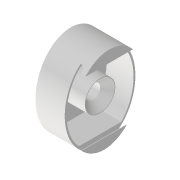
# Autodesk Inventor part: Spectrometer_pinholeholder_v0
Saved by Autodesk Inventor 2022 (Build 260153000, 153)
## iProperties
Created: 2023-02-14
Part Number: Spectrometer_pinholeholder_v0
Material: Generisch
Document SubType Name: Modeling
Designer: diederichbenedict
Density: 1 g/cm^3
Appearance: Vorgabe
Author: diederichbenedict
Autodesk Inventor part; units mm, degrees
ref_plane "YZ Plane" through (0, 0, 0) normal (1, 0, 0) x (0, 1, 0)
ref_plane "XZ Plane" through (0, 0, 0) normal (0, 1, 0) x (-1, 0, 0)
ref_plane "XY Plane" through (0, 0, 0) normal (0, 0, 1) x (1, 0, 0)
sketch "Skizze1" plane through (0, 0, 0) normal (0, 0, 1) x (1, 0, 0)
  line L0 (0, -2.5771) -> (1.4822, -3.4328)
  line L1 (-1, -2.5771) -> (0, -2.5771)
  line L2 (-1, -2.5771) -> (-1, -5.866)
  arc A0 (-1, -5.866) -> (-0.067, -6.116) centre (-0.5, -5.866) ccw
  line L3 (-0.067, -6.116) -> (1.4822, -3.4328)
  line L4 (1.6163, 54.0505) -> (2.3924, 51.1542)
  spline S0 degree 3 poles (3.0047, 50.8006) (2.979, 50.7937) (2.9516, 50.7885) (2.8832, 50.7821) (2.8365, 50.7824) (2.7601, 50.7963) (2.7337, 50.8032) (2.6799, 50.8225) (2.6525, 50.8349) (2.6004, 50.865) (2.5753, 50.8826) (2.5312, 50.9197) (2.5121, 50.9392) (2.4385, 51.0245) (2.4075, 51.0976) (2.3924, 51.1542) knots 0 0 0 0 0.142019 0.142019 0.325993 0.325993 0.417981 0.417981 0.509968 0.509968 0.59446 0.59446 0.678952 0.678952 1 1 1 1
  line L5 (3.0047, 50.8006) -> (6.1012, 51.6303)
  spline S1 degree 3 poles (1.6163, 54.0505) (1.5827, 54.1758) (1.4869, 54.2944) (1.3833, 54.3541) knots 0 0 0 0 1 1 1 1
  line L6 (26.4799, 39.8646) -> (0, 55.1528)
  line L7 (-1, 55.1528) -> (-1, 49.2)
  line L8 (-1.2, 55.3528) -> (-0.1464, 55.3528)
  line L9 (-0.1464, 55.3528) -> (1.6486, 54.3165)
  line L10 (1.6486, 54.3165) -> (2.5407, 50.9869)
  line L11 (2.7857, 50.8454) -> (6.3012, 51.7874)
  line L12 (6.3012, 51.7874) -> (6.3012, 61.3528)
  line L13 (6.3012, 61.3528) -> (-25.2, 61.3528)
  line L14 (-25.2, 61.3528) -> (-25.2, -11.866)
  line L15 (-25.2, -11.866) -> (2.1389, -11.866)
  line L16 (2.1389, -11.866) -> (2.1389, -3.4328)
  line L17 (1.7554, -3.3596) -> (0.0536, -2.3771)
  line L18 (0.0536, -2.3771) -> (-1.2, -2.3771)
  line L19 (-1.2, -2.3771) -> (-1.2, -5.866)
  arc A1 (-1.2, -5.866) -> (0.1062, -6.216) centre (-0.5, -5.866) ccw
  line L20 (0.1062, -6.216) -> (1.7554, -3.3596)
  line L21 (2.1389, -3.4328) -> (1.7554, -3.3596)
  line L22 (-1.2, -2.3771) -> (-1.2, 55.3528)
  arc A2 (2.5407, 50.9869) -> (2.7857, 50.8454) centre (2.7339, 51.0386) ccw
  point P0 (0, 0)
  point P1 (1.6852, 54.1799)
  point P2 (5.9787, 51.701)
  dimension "d0" = 0.2
  dimension "d1" = 0.2
  dimension "d3" = 0.1
  dimension "d4" = 0.1
  dimension "d5" = 0.1
  dimension "d7" = 0.2
  dimension "d8" = 6
  dimension "d9" = 24
  dimension "d10" = 6
  dimension "d26" = 0.2
  constraints: 32 end point, 5 perpendicular, 4 point on circle, 2 centre point, 2 parallel, 2 tangent, 1 horizontal, 1 vertical, 7 other
  measures "d0" distance between parallel lines of L3 L20
  measures "d1" distance from line of L7.start L8
  measures "d3" distance between parallel lines of L9 L6
  measures "d4" distance between parallel lines of L4 L10
  measures "d5" distance between parallel lines of L5 L11
  measures "d7" distance from line of L12 L5.end
  measures "d8" distance between parallel lines of L8 L13
  measures "d9" distance between parallel lines of L14 L22
  measures "d10" distance from line of L15 A0.centre
  measures "d26" radius of A2
extrude "Extrusion1" add sketch "Skizze1" along normal mid plane 60 contours L10 L9 L8 L22 L19 A1 L20 L21 L16 L15 L14 L13 L12 L11 L6 | L6 L11 A2 L10
sketch "Skizze2" plane through (-25.2, -11.866, 30) normal (-1, 0, 0) x (0, 0, 1)
  ellipse E0 centre (-30, 36.6094) end of major axis (-1.0674, 36.6094) minor radius 36.6094
  ellipse E1 centre (-30.0001, 36.9991) end of major axis (-30.0001, 6.9793) minor radius 25.9979 (-45.5397, 61.066) -> (-40.7505, 9.666) ccw projected
  line L0 (-60, 0) -> (0, 0) projected
  line L1 (0, 73.2188) -> (0, 0) projected
  line L2 (-60, 73.2188) -> (0, 73.2188) projected
  line L3 (-60, 0) -> (-60, 73.2188) projected
  point P0 (-30, 11.866)
  dimension "d27" = 73.2188
  dimension "d28" = 36.6094
  constraints: 1 centre point, 2 other
  measures "d27" distance between parallel lines of L0 L2
  measures "d28" distance from line of E0.centre L2
extrude "Extrusion2" cut sketch "Skizze2" against normal through all contours E0 keep common part
sketch "Skizze3" plane through (-1.2, 55.3528, 15.8714) normal (1, 0, 0) x (0, 0, -1)
  circle A0 centre (15.8714, -30.6094) radius 6
  ellipse E0 centre (15.8714, -30.6094) end of major axis (15.8714, 6) minor radius 28.9326 (35.3725, -3.5654) -> (-3.6296, -3.5654) ccw projected
  point P0 (15.8714, -55.3528)
  dimension "d15" = 12
  constraints: 1 centre point, 1 coincident, 1 other
  measures "d15" diameter of A0
extrude "Extrusion3" cut sketch "Skizze3" against normal blind 18
sketch "Skizze4" plane through (-19.2, 24.7434, 0) normal (1, 0, 0) x (0, 0, -1)
  circle A0 centre (0, 0) radius 6 projected
  circle A1 centre (0, 0) radius 2.9
  point P0 (0, -24.7434)
  dimension "d18" = 5.8
  constraints: 1 centre point, 1 coincident
  measures "d18" diameter of A1
extrude "Extrusion4" cut sketch "Skizze4" against normal blind 8 contours A1
chamfer "Fase1" distance 6 angle 45 1 edges at (-1.2, 24.7434, 6)
sketch "Skizze5" plane through (-25.2, 24.7434, 0) normal (-1, 0, 0) x (0, 0, 1)
  line L0 (-13.4907, 11.0031) -> (-13.4907, 11.0031) construction
  line L1 (-13.4907, 11.0031) -> (-13.4907, 11.0031) construction
  line L2 (-13.4907, 11.0031) -> (-13.4907, 11.0031) construction
  line L3 (-13.4907, 11.0031) -> (-13.4907, 11.0031) construction
  line L4 (4.984, 31.846) -> (4.984, -112.8802) construction
  line L5 (4.984, -112.8802) -> (-4.818, -112.8802) construction
  line L6 (-4.818, -112.8802) -> (-4.818, 31.846) construction
  line L7 (-4.818, 31.846) -> (4.984, 31.846) construction
  spline S0 degree 2 poles (-2.8601, 28.9674) (-2.8601, 29.7899) (-2.5163, 30.9438) (-2.2708, 31.4532) knots 0 0 0 1 2 2 2
  line L8 (-2.2708, 31.4532) -> (-1.0064, 31.4532)
  line L9 (-1.0064, 31.4532) -> (-1.0064, 31.3796)
  spline S1 degree 2 poles (-1.0064, 31.3796) (-1.4729, 30.8824) (-1.9885, 29.6242) (-1.9885, 29.0411) knots 0 0 0 1 2 2 2
  spline S2 degree 2 poles (-1.9885, 29.0411) (-1.9885, 28.2064) (-1.2949, 27.3532) (-0.7241, 27.3532) knots 0 0 0 1 2 2 2
  spline S3 degree 2 poles (-0.7241, 27.3532) (-0.2699, 27.3532) (0.2948, 27.8013) (0.4359, 28.2861) knots 0 0 0 1 2 2 2
  spline S4 degree 2 poles (0.4359, 28.2861) (0.5341, 28.636) (0.6692, 29.2191) (0.7796, 29.6549) knots 0 0 0 1 2 2 2
  spline S5 degree 2 poles (0.7796, 29.6549) (0.884, 30.0477) (1.197, 30.6676) (1.4487, 30.907) knots 0 0 0 1 2 2 2
  spline S6 degree 2 poles (1.4487, 30.907) (1.7003, 31.1402) (2.3755, 31.398) (2.8174, 31.398) knots 0 0 0 1 2 2 2
  spline S7 degree 2 poles (2.8174, 31.398) (3.738, 31.398) (4.984, 29.9618) (4.984, 28.8508) knots 0 0 0 1 2 2 2
  spline S8 degree 2 poles (4.984, 28.8508) (4.984, 28.2125) (4.7324, 27.0831) (4.493, 26.5983) knots 0 0 0 1 2 2 2
  line L10 (4.493, 26.5983) -> (3.29, 26.5983)
  line L11 (3.29, 26.5983) -> (3.29, 26.6719)
  spline S9 degree 2 poles (3.29, 26.6719) (3.6214, 27.034) (4.1124, 28.1634) (4.1124, 28.7833) knots 0 0 0 1 2 2 2
  spline S10 degree 2 poles (4.1124, 28.7833) (4.1124, 29.483) (3.4557, 30.3484) (2.9217, 30.3484) knots 0 0 0 1 2 2 2
  spline S11 degree 2 poles (2.9217, 30.3484) (2.443, 30.3484) (1.8722, 29.839) (1.7433, 29.3603) knots 0 0 0 1 2 2 2
  spline S12 degree 2 poles (1.7433, 29.3603) (1.6573, 29.0411) (1.4364, 28.1143) (1.3443, 27.8074) knots 0 0 0 1 2 2 2
  spline S13 degree 2 poles (1.3443, 27.8074) (1.1049, 27.0279) (0.1413, 26.3036) (-0.5645, 26.3036) knots 0 0 0 1 2 2 2
  spline S14 degree 2 poles (-0.5645, 26.3036) (-1.0126, 26.3036) (-1.8719, 26.6658) (-2.1726, 26.9911) knots 0 0 0 1 2 2 2
  spline S15 degree 2 poles (-2.1726, 26.9911) (-2.5041, 27.3532) (-2.8601, 28.2739) (-2.8601, 28.9674) knots 0 0 0 1 2 2 2
  spline S16 degree 2 poles (0.2702, 20.5894) (-1.1538, 20.5894) (-2.8355, 21.9458) (-2.8355, 22.9831) knots 0 0 0 1 2 2 2
  spline S17 degree 2 poles (-2.8355, 22.9831) (-2.8355, 23.4066) (-2.6391, 24.0572) (-2.4365, 24.3948) knots 0 0 0 1 2 2 2
  line L12 (-2.4365, 24.3948) -> (-4.818, 24.3948)
  line L13 (-4.818, 24.3948) -> (-4.818, 25.3523)
  line L14 (-4.818, 25.3523) -> (2.9585, 25.3523)
  line L15 (2.9585, 25.3523) -> (2.9585, 24.3948)
  line L16 (2.9585, 24.3948) -> (2.3632, 24.3948)
  spline S18 degree 2 poles (2.3632, 24.3948) (2.6885, 24.0388) (3.1181, 23.1673) (3.1181, 22.6578) knots 0 0 0 1 2 2 2
  spline S19 degree 2 poles (3.1181, 22.6578) (3.1181, 21.6819) (1.5714, 20.5894) (0.2702, 20.5894) knots 0 0 0 1 2 2 2
  spline S20 degree 2 poles (0.1597, 21.5776) (1.1356, 21.5776) (2.2097, 22.1975) (2.2097, 22.8911) knots 0 0 0 1 2 2 2
  spline S21 degree 2 poles (2.2097, 22.8911) (2.2097, 23.2961) (1.8476, 24.0572) (1.5653, 24.3948) knots 0 0 0 1 2 2 2
  line L17 (1.5653, 24.3948) -> (-1.6632, 24.3948)
  spline S22 degree 2 poles (-1.6632, 24.3948) (-1.8412, 24.0204) (-1.9762, 23.4864) (-1.9762, 23.1427) knots 0 0 0 1 2 2 2
  spline S23 degree 2 poles (-1.9762, 23.1427) (-1.9762, 22.4) (-0.8837, 21.5776) (0.1597, 21.5776) knots 0 0 0 1 2 2 2
  spline S24 degree 2 poles (-2.8539, 17.1277) (-2.8539, 18.4903) (-1.3256, 19.9879) (0.0861, 19.9879) knots 0 0 0 1 2 2 2
  spline S25 degree 2 poles (0.0861, 19.9879) (1.4732, 19.9879) (3.1181, 18.5332) (3.1181, 17.3609) knots 0 0 0 1 2 2 2
  spline S26 degree 2 poles (3.1181, 17.3609) (3.1181, 16.8331) (2.8112, 16.0168) (2.4859, 15.716) knots 0 0 0 1 2 2 2
  spline S27 degree 2 poles (2.4859, 15.716) (2.1606, 15.4091) (1.2216, 15.0838) (0.5403, 15.0838) knots 0 0 0 1 2 2 2
  line L18 (0.5403, 15.0838) -> (0.0186, 15.0838)
  line L19 (0.0186, 15.0838) -> (0.0186, 19.0181)
  spline S28 degree 2 poles (0.0186, 19.0181) (-0.9696, 19.0181) (-2.0192, 18.0238) (-2.0192, 17.14) knots 0 0 0 1 2 2 2
  spline S29 degree 2 poles (-2.0192, 17.14) (-2.0192, 16.8269) (-1.878, 16.2193) (-1.7675, 15.9738) knots 0 0 0 1 2 2 2
  spline S30 degree 2 poles (-1.7675, 15.9738) (-1.6448, 15.716) (-1.43, 15.36) (-1.3318, 15.2434) knots 0 0 0 1 2 2 2
  line L20 (-1.3318, 15.2434) -> (-1.3318, 15.1882)
  line L21 (-1.3318, 15.1882) -> (-2.3752, 15.1882)
  spline S31 degree 2 poles (-2.3752, 15.1882) (-2.4427, 15.3539) (-2.6391, 15.8572) (-2.6943, 16.0536) knots 0 0 0 1 2 2 2
  spline S32 degree 2 poles (-2.6943, 16.0536) (-2.7741, 16.3298) (-2.8539, 16.784) (-2.8539, 17.1277) knots 0 0 0 1 2 2 2
  spline S33 degree 2 poles (0.749, 16.0168) (1.1356, 16.029) (1.7003, 16.1886) (1.8906, 16.3421) knots 0 0 0 1 2 2 2
  spline S34 degree 2 poles (1.8906, 16.3421) (2.1054, 16.5078) (2.3325, 17.0295) (2.3325, 17.4162) knots 0 0 0 1 2 2 2
  spline S35 degree 2 poles (2.3325, 17.4162) (2.3325, 17.7967) (2.1054, 18.3307) (1.8844, 18.5517) knots 0 0 0 1 2 2 2
  spline S36 degree 2 poles (1.8844, 18.5517) (1.6573, 18.7665) (1.1111, 18.9874) (0.749, 19.0181) knots 0 0 0 1 2 2 2
  line L22 (0.749, 19.0181) -> (0.749, 16.0168)
  spline S37 degree 2 poles (-2.8539, 11.8554) (-2.8539, 12.4446) (-2.4918, 13.4205) (-2.1235, 13.7703) knots 0 0 0 1 2 2 2
  spline S38 degree 2 poles (-2.1235, 13.7703) (-1.7614, 14.1202) (-0.6443, 14.5069) (0.1045, 14.5069) knots 0 0 0 1 2 2 2
  spline S39 degree 2 poles (0.1045, 14.5069) (0.8533, 14.5069) (1.9458, 14.1079) (2.3141, 13.7703) knots 0 0 0 1 2 2 2
  spline S40 degree 2 poles (2.3141, 13.7703) (2.6885, 13.4328) (3.0874, 12.4323) (3.0874, 11.8554) knots 0 0 0 1 2 2 2
  spline S41 degree 2 poles (3.0874, 11.8554) (3.0874, 11.3889) (2.8235, 10.5173) (2.6517, 10.1797) knots 0 0 0 1 2 2 2
  line L23 (2.6517, 10.1797) -> (1.5775, 10.1797)
  line L24 (1.5775, 10.1797) -> (1.5775, 10.235)
  spline S42 degree 2 poles (1.5775, 10.235) (1.6635, 10.3393) (1.8844, 10.6585) (2.0011, 10.8856) knots 0 0 0 1 2 2 2
  spline S43 degree 2 poles (2.0011, 10.8856) (2.0993, 11.0881) (2.2527, 11.6283) (2.2527, 11.8738) knots 0 0 0 1 2 2 2
  spline S44 degree 2 poles (2.2527, 11.8738) (2.2527, 12.6164) (1.1295, 13.5187) (0.1045, 13.5187) knots 0 0 0 1 2 2 2
  spline S45 degree 2 poles (0.1045, 13.5187) (-0.896, 13.5187) (-2.0192, 12.6471) (-2.0192, 11.8738) knots 0 0 0 1 2 2 2
  spline S46 degree 2 poles (-2.0192, 11.8738) (-2.0192, 11.4073) (-1.6325, 10.5603) (-1.3318, 10.235) knots 0 0 0 1 2 2 2
  line L25 (-1.3318, 10.235) -> (-1.3318, 10.1797)
  line L26 (-1.3318, 10.1797) -> (-2.4059, 10.1797)
  spline S47 degree 2 poles (-2.4059, 10.1797) (-2.4734, 10.3209) (-2.6636, 10.7506) (-2.7066, 10.9224) knots 0 0 0 1 2 2 2
  spline S48 degree 2 poles (-2.7066, 10.9224) (-2.7803, 11.1679) (-2.8539, 11.5546) (-2.8539, 11.8554) knots 0 0 0 1 2 2 2
  spline S49 degree 2 poles (-2.8355, 7.5896) (-2.8355, 8.3691) (-1.9455, 9.2468) (-0.9819, 9.2468) knots 0 0 0 1 2 2 2
  line L27 (-0.9819, 9.2468) -> (2.1668, 9.2468)
  line L28 (2.1668, 9.2468) -> (2.1668, 9.8913)
  line L29 (2.1668, 9.8913) -> (2.9585, 9.8913)
  line L30 (2.9585, 9.8913) -> (2.9585, 9.2468)
  line L31 (2.9585, 9.2468) -> (4.5912, 9.2468)
  line L32 (4.5912, 9.2468) -> (4.5912, 8.2893)
  line L33 (4.5912, 8.2893) -> (2.9585, 8.2893)
  line L34 (2.9585, 8.2893) -> (2.9585, 6.5278)
  line L35 (2.9585, 6.5278) -> (2.1668, 6.5278)
  line L36 (2.1668, 6.5278) -> (2.1668, 8.2893)
  line L37 (2.1668, 8.2893) -> (-0.54, 8.2893)
  spline S50 degree 2 poles (-0.54, 8.2893) (-0.9696, 8.2893) (-1.4422, 8.2586) (-1.6448, 8.1543) knots 0 0 0 1 2 2 2
  spline S51 degree 2 poles (-1.6448, 8.1543) (-1.8228, 8.0684) (-2.0008, 7.6817) (-2.0008, 7.3502) knots 0 0 0 1 2 2 2
  spline S52 degree 2 poles (-2.0008, 7.3502) (-2.0008, 7.117) (-1.8596, 6.6812) (-1.8166, 6.583) knots 0 0 0 1 2 2 2
  line L38 (-1.8166, 6.583) -> (-1.8166, 6.5278)
  line L39 (-1.8166, 6.5278) -> (-2.6759, 6.5278)
  spline S53 degree 2 poles (-2.6759, 6.5278) (-2.7496, 6.7978) (-2.8355, 7.3502) (-2.8355, 7.5896) knots 0 0 0 1 2 2 2
  line L40 (1.9335, 2.8083) -> (1.9335, 2.8574)
  spline S54 degree 2 poles (1.9335, 2.8574) (1.9642, 2.9679) (1.9765, 3.2072) (1.9765, 3.373) knots 0 0 0 1 2 2 2
  spline S55 degree 2 poles (1.9765, 3.373) (1.9765, 3.7596) (1.6389, 4.5207) (1.3075, 4.8644) knots 0 0 0 1 2 2 2
  line L41 (1.3075, 4.8644) -> (-2.725, 4.8644)
  line L42 (-2.725, 4.8644) -> (-2.725, 5.8219)
  line L43 (-2.725, 5.8219) -> (2.9585, 5.8219)
  line L44 (2.9585, 5.8219) -> (2.9585, 4.8644)
  line L45 (2.9585, 4.8644) -> (2.1115, 4.8644)
  spline S56 degree 2 poles (2.1115, 4.8644) (2.578, 4.3427) (2.9585, 3.5632) (2.9585, 3.195) knots 0 0 0 1 2 2 2
  spline S57 degree 2 poles (2.9585, 3.195) (2.9585, 3.0477) (2.9463, 2.9004) (2.9279, 2.8083) knots 0 0 0 1 2 2 2
  line L46 (2.9279, 2.8083) -> (1.9335, 2.8083)
  spline S58 degree 2 poles (0.1168, -2.6052) (-1.3195, -2.6052) (-2.8846, -1.2242) (-2.8846, -0.0703) knots 0 0 0 1 2 2 2
  spline S59 degree 2 poles (-2.8846, -0.0703) (-2.8846, 1.1143) (-1.2704, 2.4707) (0.1168, 2.4707) knots 0 0 0 1 2 2 2
  spline S60 degree 2 poles (0.1168, 2.4707) (1.5407, 2.4707) (3.1181, 1.0713) (3.1181, -0.0703) knots 0 0 0 1 2 2 2
  spline S61 degree 2 poles (3.1181, -0.0703) (3.1181, -1.2242) (1.5469, -2.6052) (0.1168, -2.6052) knots 0 0 0 1 2 2 2
  spline S62 degree 2 poles (0.1168, -1.617) (1.2216, -1.617) (2.2957, -0.813) (2.2957, -0.0703) knots 0 0 0 1 2 2 2
  spline S63 degree 2 poles (2.2957, -0.0703) (2.2957, 0.6723) (1.2216, 1.4825) (0.1168, 1.4825) knots 0 0 0 1 2 2 2
  spline S64 degree 2 poles (0.1168, 1.4825) (-0.9573, 1.4825) (-2.0621, 0.6723) (-2.0621, -0.0703) knots 0 0 0 1 2 2 2
  spline S65 degree 2 poles (-2.0621, -0.0703) (-2.0621, -0.8069) (-0.9758, -1.617) (0.1168, -1.617) knots 0 0 0 1 2 2 2
  line L47 (-2.725, -10.0319) -> (0.5648, -10.0319)
  spline S66 degree 2 poles (0.5648, -10.0319) (0.9576, -10.0319) (1.6267, -9.9705) (1.8108, -9.8723) knots 0 0 0 1 2 2 2
  spline S67 degree 2 poles (1.8108, -9.8723) (2.0133, -9.7741) (2.2097, -9.3997) (2.2097, -9.0744) knots 0 0 0 1 2 2 2
  spline S68 degree 2 poles (2.2097, -9.0744) (2.2097, -8.7798) (1.8476, -8.1047) (1.5039, -7.7487) knots 0 0 0 1 2 2 2
  spline S69 degree 2 poles (1.5039, -7.7487) (1.418, -7.7548) (1.1786, -7.7671) (1.019, -7.7671) knots 0 0 0 1 2 2 2
  line L48 (1.019, -7.7671) -> (-2.725, -7.7671)
  line L49 (-2.725, -7.7671) -> (-2.725, -6.8096)
  line L50 (-2.725, -6.8096) -> (0.5648, -6.8096)
  spline S70 degree 2 poles (0.5648, -6.8096) (0.9576, -6.8096) (1.6267, -6.7482) (1.8108, -6.65) knots 0 0 0 1 2 2 2
  spline S71 degree 2 poles (1.8108, -6.65) (2.0133, -6.5518) (2.2097, -6.1774) (2.2097, -5.8521) knots 0 0 0 1 2 2 2
  spline S72 degree 2 poles (2.2097, -5.8521) (2.2097, -5.5452) (1.8231, -4.8639) (1.5223, -4.5447) knots 0 0 0 1 2 2 2
  line L51 (1.5223, -4.5447) -> (-2.725, -4.5447)
  line L52 (-2.725, -4.5447) -> (-2.725, -3.5873)
  line L53 (-2.725, -3.5873) -> (2.9585, -3.5873)
  line L54 (2.9585, -3.5873) -> (2.9585, -4.5447)
  line L55 (2.9585, -4.5447) -> (2.3325, -4.5447)
  spline S73 degree 2 poles (2.3325, -4.5447) (2.7069, -4.9192) (3.1181, -5.6557) (3.1181, -6.0976) knots 0 0 0 1 2 2 2
  spline S74 degree 2 poles (3.1181, -6.0976) (3.1181, -6.6009) (2.6578, -7.3804) (2.1361, -7.5829) knots 0 0 0 1 2 2 2
  spline S75 degree 2 poles (2.1361, -7.5829) (2.621, -8.0187) (3.1181, -8.8412) (3.1181, -9.3199) knots 0 0 0 1 2 2 2
  spline S76 degree 2 poles (3.1181, -9.3199) (3.1181, -9.6882) (2.891, -10.2897) (2.6332, -10.5107) knots 0 0 0 1 2 2 2
  spline S77 degree 2 poles (2.6332, -10.5107) (2.3755, -10.7378) (1.6021, -10.9894) (1.019, -10.9894) knots 0 0 0 1 2 2 2
  line L56 (1.019, -10.9894) -> (-2.725, -10.9894)
  line L57 (-2.725, -10.9894) -> (-2.725, -10.0319)
  spline S78 degree 2 poles (-2.8539, -14.801) (-2.8539, -13.4384) (-1.3256, -11.9408) (0.0861, -11.9408) knots 0 0 0 1 2 2 2
  spline S79 degree 2 poles (0.0861, -11.9408) (1.4732, -11.9408) (3.1181, -13.3954) (3.1181, -14.5677) knots 0 0 0 1 2 2 2
  spline S80 degree 2 poles (3.1181, -14.5677) (3.1181, -15.0956) (2.8112, -15.9119) (2.4859, -16.2126) knots 0 0 0 1 2 2 2
  spline S81 degree 2 poles (2.4859, -16.2126) (2.1606, -16.5195) (1.2216, -16.8448) (0.5403, -16.8448) knots 0 0 0 1 2 2 2
  line L58 (0.5403, -16.8448) -> (0.0186, -16.8448)
  line L59 (0.0186, -16.8448) -> (0.0186, -12.9105)
  spline S82 degree 2 poles (0.0186, -12.9105) (-0.9696, -12.9105) (-2.0192, -13.9048) (-2.0192, -14.7887) knots 0 0 0 1 2 2 2
  spline S83 degree 2 poles (-2.0192, -14.7887) (-2.0192, -15.1017) (-1.878, -15.7093) (-1.7675, -15.9549) knots 0 0 0 1 2 2 2
  spline S84 degree 2 poles (-1.7675, -15.9549) (-1.6448, -16.2126) (-1.43, -16.5686) (-1.3318, -16.6852) knots 0 0 0 1 2 2 2
  line L60 (-1.3318, -16.6852) -> (-1.3318, -16.7405)
  line L61 (-1.3318, -16.7405) -> (-2.3752, -16.7405)
  spline S85 degree 2 poles (-2.3752, -16.7405) (-2.4427, -16.5748) (-2.6391, -16.0715) (-2.6943, -15.8751) knots 0 0 0 1 2 2 2
  spline S86 degree 2 poles (-2.6943, -15.8751) (-2.7741, -15.5989) (-2.8539, -15.1447) (-2.8539, -14.801) knots 0 0 0 1 2 2 2
  spline S87 degree 2 poles (0.749, -15.9119) (1.1356, -15.8996) (1.7003, -15.74) (1.8906, -15.5866) knots 0 0 0 1 2 2 2
  spline S88 degree 2 poles (1.8906, -15.5866) (2.1054, -15.4209) (2.3325, -14.8992) (2.3325, -14.5125) knots 0 0 0 1 2 2 2
  spline S89 degree 2 poles (2.3325, -14.5125) (2.3325, -14.1319) (2.1054, -13.5979) (1.8844, -13.377) knots 0 0 0 1 2 2 2
  spline S90 degree 2 poles (1.8844, -13.377) (1.6573, -13.1622) (1.1111, -12.9412) (0.749, -12.9105) knots 0 0 0 1 2 2 2
  line L62 (0.749, -12.9105) -> (0.749, -15.9119)
  spline S91 degree 2 poles (-2.8355, -19.5332) (-2.8355, -18.7537) (-1.9455, -17.876) (-0.9819, -17.876) knots 0 0 0 1 2 2 2
  line L63 (-0.9819, -17.876) -> (2.1668, -17.876)
  line L64 (2.1668, -17.876) -> (2.1668, -17.2315)
  line L65 (2.1668, -17.2315) -> (2.9585, -17.2315)
  line L66 (2.9585, -17.2315) -> (2.9585, -17.876)
  line L67 (2.9585, -17.876) -> (4.5912, -17.876)
  line L68 (4.5912, -17.876) -> (4.5912, -18.8335)
  line L69 (4.5912, -18.8335) -> (2.9585, -18.8335)
  line L70 (2.9585, -18.8335) -> (2.9585, -20.595)
  line L71 (2.9585, -20.595) -> (2.1668, -20.595)
  line L72 (2.1668, -20.595) -> (2.1668, -18.8335)
  line L73 (2.1668, -18.8335) -> (-0.54, -18.8335)
  spline S92 degree 2 poles (-0.54, -18.8335) (-0.9696, -18.8335) (-1.4422, -18.8642) (-1.6448, -18.9685) knots 0 0 0 1 2 2 2
  spline S93 degree 2 poles (-1.6448, -18.9685) (-1.8228, -19.0544) (-2.0008, -19.4411) (-2.0008, -19.7725) knots 0 0 0 1 2 2 2
  spline S94 degree 2 poles (-2.0008, -19.7725) (-2.0008, -20.0058) (-1.8596, -20.4416) (-1.8166, -20.5398) knots 0 0 0 1 2 2 2
  line L74 (-1.8166, -20.5398) -> (-1.8166, -20.595)
  line L75 (-1.8166, -20.595) -> (-2.6759, -20.595)
  spline S95 degree 2 poles (-2.6759, -20.595) (-2.7496, -20.3249) (-2.8355, -19.7725) (-2.8355, -19.5332) knots 0 0 0 1 2 2 2
  spline S96 degree 2 poles (-2.8539, -23.7682) (-2.8539, -22.4056) (-1.3256, -20.908) (0.0861, -20.908) knots 0 0 0 1 2 2 2
  spline S97 degree 2 poles (0.0861, -20.908) (1.4732, -20.908) (3.1181, -22.3627) (3.1181, -23.535) knots 0 0 0 1 2 2 2
  spline S98 degree 2 poles (3.1181, -23.535) (3.1181, -24.0628) (2.8112, -24.8792) (2.4859, -25.1799) knots 0 0 0 1 2 2 2
  spline S99 degree 2 poles (2.4859, -25.1799) (2.1606, -25.4868) (1.2216, -25.8121) (0.5403, -25.8121) knots 0 0 0 1 2 2 2
  line L76 (0.5403, -25.8121) -> (0.0186, -25.8121)
  line L77 (0.0186, -25.8121) -> (0.0186, -21.8778)
  spline S100 degree 2 poles (0.0186, -21.8778) (-0.9696, -21.8778) (-2.0192, -22.8721) (-2.0192, -23.7559) knots 0 0 0 1 2 2 2
  spline S101 degree 2 poles (-2.0192, -23.7559) (-2.0192, -24.069) (-1.878, -24.6766) (-1.7675, -24.9221) knots 0 0 0 1 2 2 2
  spline S102 degree 2 poles (-1.7675, -24.9221) (-1.6448, -25.1799) (-1.43, -25.5359) (-1.3318, -25.6525) knots 0 0 0 1 2 2 2
  line L78 (-1.3318, -25.6525) -> (-1.3318, -25.7078)
  line L79 (-1.3318, -25.7078) -> (-2.3752, -25.7078)
  spline S103 degree 2 poles (-2.3752, -25.7078) (-2.4427, -25.542) (-2.6391, -25.0387) (-2.6943, -24.8423) knots 0 0 0 1 2 2 2
  spline S104 degree 2 poles (-2.6943, -24.8423) (-2.7741, -24.5661) (-2.8539, -24.1119) (-2.8539, -23.7682) knots 0 0 0 1 2 2 2
  spline S105 degree 2 poles (0.749, -24.8792) (1.1356, -24.8669) (1.7003, -24.7073) (1.8906, -24.5539) knots 0 0 0 1 2 2 2
  spline S106 degree 2 poles (1.8906, -24.5539) (2.1054, -24.3881) (2.3325, -23.8664) (2.3325, -23.4797) knots 0 0 0 1 2 2 2
  spline S107 degree 2 poles (2.3325, -23.4797) (2.3325, -23.0992) (2.1054, -22.5652) (1.8844, -22.3443) knots 0 0 0 1 2 2 2
  spline S108 degree 2 poles (1.8844, -22.3443) (1.6573, -22.1294) (1.1111, -21.9085) (0.749, -21.8778) knots 0 0 0 1 2 2 2
  line L80 (0.749, -21.8778) -> (0.749, -24.8792)
  line L81 (1.9335, -29.7955) -> (1.9335, -29.7464)
  spline S109 degree 2 poles (1.9335, -29.7464) (1.9642, -29.6359) (1.9765, -29.3966) (1.9765, -29.2308) knots 0 0 0 1 2 2 2
  spline S110 degree 2 poles (1.9765, -29.2308) (1.9765, -28.8442) (1.6389, -28.0831) (1.3075, -27.7394) knots 0 0 0 1 2 2 2
  line L82 (1.3075, -27.7394) -> (-2.725, -27.7394)
  line L83 (-2.725, -27.7394) -> (-2.725, -26.7819)
  line L84 (-2.725, -26.7819) -> (2.9585, -26.7819)
  line L85 (2.9585, -26.7819) -> (2.9585, -27.7394)
  line L86 (2.9585, -27.7394) -> (2.1115, -27.7394)
  spline S111 degree 2 poles (2.1115, -27.7394) (2.578, -28.2611) (2.9585, -29.0406) (2.9585, -29.4088) knots 0 0 0 1 2 2 2
  spline S112 degree 2 poles (2.9585, -29.4088) (2.9585, -29.5561) (2.9463, -29.7034) (2.9279, -29.7955) knots 0 0 0 1 2 2 2
  line L87 (2.9279, -29.7955) -> (1.9335, -29.7955)
  point P0 (0, -24.7434)
  constraints: 4 other
extrude "Extrusion5" cut sketch "Skizze5" against normal blind 1
sketch "Skizze6" plane through (-1.2, 55.3528, 15.8714) normal (1, 0, 0) x (0, 0, -1)
  ellipse E0 centre (15.8714, -30.6094) end of major axis (15.8714, 6) minor radius 28.9326 (31.7429, -61.2188) -> (31.7429, 0) ccw projected
  line L0 (31.7429, 0) -> (0, 0) projected
  ellipse E1 centre (15.8714, -30.6094) end of major axis (15.8714, 6) minor radius 28.9326 (0, 0) -> (0, -61.2188) ccw projected
  line L1 (31.7429, -61.2188) -> (0, -61.2188) projected
  circle A0 centre (15.8714, -30.6094) radius 12 projected
  line L2 (0.5495, -1.5) -> (31.1934, -1.5)
  line L3 (31.1934, -59.7188) -> (0.5495, -59.7188)
  circle A1 centre (15.8714, -30.6094) radius 12.5
  line L4 (-3.0365, -5.1887) -> (34.7794, -5.1887)
  line L5 (-1.5046, -57.7622) -> (33.2474, -57.7622)
  spline S0 degree 5 poles (0.5495, -59.7189) (-1.0101, -58.3731) (-2.4469, -56.8848) (-3.7539, -55.2809) (-7.4701, -49.9316) (-9.9154, -43.8286) (-11.0118, -39.4835) (-12.1107, -30.6094) (-11.0118, -21.7354) (-9.9154, -17.3903) (-7.4701, -11.2872) (-3.7539, -5.9379) (-2.4469, -4.334) (-1.0101, -2.8457) (0.5495, -1.5) knots 0 0 0 0 0 0 0.158539 0.158539 0.158539 0.5 0.5 0.5 0.841461 0.841461 0.841461 1 1 1 1 1 1
  spline S1 degree 5 poles (31.1934, -1.5) (32.753, -2.8457) (34.1898, -4.334) (35.4968, -5.9379) (39.213, -11.2872) (41.6583, -17.3903) (42.7546, -21.7354) (43.8536, -30.6094) (42.7546, -39.4835) (41.6583, -43.8286) (39.213, -49.9316) (35.4968, -55.2809) (34.1898, -56.8848) (32.753, -58.3731) (31.1934, -59.7189) knots 0 0 0 0 0 0 0.158539 0.158539 0.158539 0.5 0.5 0.5 0.841461 0.841461 0.841461 1 1 1 1 1 1
  point P0 (15.8714, -55.3528)
  dimension "d30" = 1.5
  dimension "d31" = 0.5
  constraints: 8 end point, 4 parallel, 1 centre point, 1 horizontal, 12 other
  measures "d31" radial gap between concentric circles of A0 A1
extrude "Extrusion6" cut sketch "Skizze6" against normal blind 22 contours L2 S1 L4 S0 | L4 S1 L5 S0
equation "\"d28\" = 0.5 * d27"
